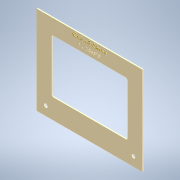
# Autodesk Inventor part: front
Saved by Autodesk Inventor 2022 (Build 260153000, 153)
## iProperties
Created: 2023-08-31
Part Number: front
Material: Generic
Document SubType Name: Modeling
Designer: THK
Density: 1 g/cm^3
Appearance: Red
Author: THK
Autodesk Inventor part; units mm, degrees
ref_plane "YZ Plane" through (0, 0, 0) normal (1, 0, 0) x (0, 1, 0)
ref_plane "XZ Plane" through (0, 0, 0) normal (0, 1, 0) x (-1, 0, 0)
ref_plane "XY Plane" through (0, 0, 0) normal (0, 0, 1) x (1, 0, 0)
sketch "Sketch1" plane through (0, 0, 0) normal (0, 0, 1) x (1, 0, 0)
  line L0 (-264.1156, 220.8859) -> (264.1156, 220.8859)
  line L1 (264.1156, 220.8859) -> (264.1156, -220.8859)
  line L2 (264.1156, -220.8859) -> (-264.1156, -220.8859)
  line L3 (-264.1156, -220.8859) -> (-264.1156, 220.8859)
  line L4 (-264.1156, 220.8859) -> (264.1156, -220.8859) construction
  line L5 (264.1156, 220.8859) -> (-264.1156, -220.8859) construction
  point P0 (0, 0)
  dimension "d0" = 528.2313
  dimension "d1" = 441.7719
  constraints: 12 end point, 2 midpoint, 2 parallel, 1 horizontal, 1 perpendicular
  measures "d0" distance of L1.end L2.end
  measures "d1" distance of L0.end L1.end
extrude "Extrusion1" add sketch "Sketch1" against normal blind 6
sketch "Sketch2" plane through (0, 0, 0) normal (0, 0, 1) x (1, 0, 0)
  line L0 (-181.2094, 146.2703) -> (181.2094, 146.2703)
  line L1 (189.5, 137.9797) -> (189.5, -113.1078)
  line L2 (181.2094, -121.3984) -> (-181.2094, -121.3984)
  line L3 (-189.5, -113.1078) -> (-189.5, 137.9797)
  line L4 (-189.5, 146.2703) -> (189.5, -121.3984) construction
  line L5 (189.5, 146.2703) -> (-189.5, -121.3984) construction
  line L6 (189.5, 105.3059) -> (264.1156, 105.3059) construction
  line L7 (264.1156, 220.8859) -> (264.1156, -220.8859) projected
  line L8 (72.6661, 146.2703) -> (72.6661, 220.8859) construction
  line L9 (-264.1156, 220.8859) -> (264.1156, 220.8859) projected
  arc A0 (-181.2094, 146.2703) -> (-189.5, 137.9797) centre (-181.2094, 137.9797) ccw
  arc A1 (189.5, 137.9797) -> (181.2094, 146.2703) centre (181.2094, 137.9797) ccw
  arc A2 (181.2094, -121.3984) -> (189.5, -113.1078) centre (181.2094, -113.1078) ccw
  arc A3 (-189.5, -113.1078) -> (-181.2094, -121.3984) centre (-181.2094, -113.1078) ccw
  point P0 (0, 0)
  point P1 (0, 12.4359)
  point P2 (0, 12.4359)
  dimension "d4" = 267.6687
  dimension "d5" = 379
  dimension "d6" = 74.6156
  dimension "d7" = 8.2906
  constraints: 16 end point, 12 point on line, 8 point on circle, 8 tangent, 4 centre point, 3 equal radius, 3 midpoint, 2 horizontal, 2 parallel, 2 perpendicular, 1 vertical, 1 vertical alignment
  measures "d4" distance between parallel lines of L2 L0
  measures "d5" distance between parallel lines of L1 L3
  measures "d6" distance between parallel lines of L7 L1
  measures "d7" radius of A0
extrude "Extrusion2" cut sketch "Sketch2" against normal through all
sketch "Sketch3" plane through (0, 0, 0) normal (0, 0, 1) x (1, 0, 0)
  line L0 (-264.1156, -220.8859) -> (-264.1156, 220.8859) construction
  line L1 (-264.1156, -220.8859) -> (-219.1094, -220.8859) construction
  line L2 (-219.1094, -220.8859) -> (-219.1094, -175.8797) construction
  line L3 (-219.1094, -175.8797) -> (-264.1156, -175.8797) construction
  line L4 (-264.1156, -175.8797) -> (-264.1156, -220.8859) construction
  point P0 (0, 0)
  dimension "d10" = 45.0063
  dimension "d11" = 45.0063
  constraints: 8 end point, 2 parallel, 1 coincident, 1 horizontal, 1 perpendicular
  measures "d10" distance of L3.end L2.end
  measures "d11" distance of L2.end L1.end
hole "Hole1" at (-219.1094, -175.8797, 0) direction (0, 0, -1) diameter 19 end through all
mirror "Mirror1" about plane through (0, 0, 0) normal (1, 0, 0) of "Hole1"
sketch "Sketch4" plane through (0, 0, 0) normal (0, 0, 1) x (1, 0, 0)
  line L0 (-184.2304, 215.2203) -> (184.2304, 215.2203) construction
  line L1 (184.2304, 215.2203) -> (184.2304, 133.9272) construction
  line L2 (184.2304, 133.9272) -> (-184.2304, 133.9272) construction
  line L3 (-184.2304, 133.9272) -> (-184.2304, 215.2203) construction
  spline S0 degree 2 poles (-80.6136, 205.9581) (-79.2403, 205.9581) (-73.7327, 205.7536) (-72.3594, 205.7536) knots 0 0 0 1 2 2 2
  spline S1 degree 2 poles (-72.3594, 205.7536) (-70.2264, 205.7536) (-69.4668, 205.8558) knots 0 0 0 1 1 1
  spline S2 degree 2 poles (-69.4668, 205.8558) (-67.8159, 206.0896) (-66.8663, 206.9661) knots 0 0 0 1 1 1
  spline S3 degree 2 poles (-66.8663, 206.9661) (-67.4653, 204.8916) (-69.8904, 203.7813) knots 0 0 0 1 1 1
  spline S4 degree 2 poles (-69.8904, 203.7813) (-70.8693, 203.3285) (-72.4178, 203.3285) knots 0 0 0 1 1 1
  spline S5 degree 2 poles (-72.4178, 203.3285) (-72.7392, 203.3285) (-75.3105, 203.3869) knots 0 0 0 1 1 1
  line L4 (-75.3105, 203.3869) -> (-78.2177, 203.3869)
  spline S6 degree 2 poles (-78.2177, 203.3869) (-78.5829, 203.3869) (-79.9562, 203.3285) knots 0 0 0 1 1 1
  spline S7 degree 2 poles (-79.9562, 203.3285) (-79.8247, 202.4665) (-78.8459, 201.327) knots 0 0 0 1 1 1
  spline S8 degree 2 poles (-78.8459, 201.327) (-77.3703, 199.6031) (-72.8707, 197.5578) (-70.5479, 197.5578) knots 0 0 0 1 2 2 2
  spline S9 degree 2 poles (-70.5479, 197.5578) (-68.7801, 197.5578) (-64.3389, 198.9895) (-63.0095, 200.0122) knots 0 0 0 1 2 2 2
  spline S10 degree 2 poles (-63.0095, 200.0122) (-63.4624, 199.121) (-64.485, 198.2445) knots 0 0 0 1 1 1
  spline S11 degree 2 poles (-64.485, 198.2445) (-66.092, 196.9004) (-70.4748, 195.3226) (-72.6224, 195.3226) knots 0 0 0 1 2 2 2
  spline S12 degree 2 poles (-72.6224, 195.3226) (-74.1855, 195.3226) (-77.9255, 196.5352) (-79.1088, 197.4848) knots 0 0 0 1 2 2 2
  spline S13 degree 2 poles (-79.1088, 197.4848) (-80.3945, 198.5074) (-82.2498, 201.7507) (-82.5128, 203.4161) knots 0 0 0 1 2 2 2
  spline S14 degree 2 poles (-82.5128, 203.4161) (-83.7984, 203.3577) (-84.2513, 203.3285) knots 0 0 0 1 1 1
  spline S15 degree 2 poles (-84.2513, 203.3285) (-85.1717, 203.2554) (-85.9313, 202.9924) knots 0 0 0 1 1 1
  spline S16 degree 2 poles (-85.9313, 202.9924) (-84.8795, 205.2861) (-82.2644, 205.8851) knots 0 0 0 1 1 1
  spline S17 degree 2 poles (-82.2644, 205.8851) (-81.4463, 209.7419) (-78.9481, 211.9041) knots 0 0 0 1 1 1
  spline S18 degree 2 poles (-78.9481, 211.9041) (-77.1658, 213.4526) (-72.2279, 215.2203) (-69.8174, 215.2203) knots 0 0 0 1 2 2 2
  spline S19 degree 2 poles (-69.8174, 215.2203) (-67.3923, 215.2203) (-65.4638, 214.5045) knots 0 0 0 1 1 1
  spline S20 degree 2 poles (-65.4638, 214.5045) (-62.7758, 213.5403) (-62.7758, 211.5096) knots 0 0 0 1 1 1
  spline S21 degree 2 poles (-62.7758, 211.5096) (-62.7758, 209.8442) (-64.3389, 207.682) knots 0 0 0 1 1 1
  spline S22 degree 2 poles (-64.3389, 207.682) (-64.2805, 209.6104) (-65.9898, 211.8164) (-67.889, 212.43) knots 0 0 0 1 2 2 2
  spline S23 degree 2 poles (-67.889, 212.43) (-69.5544, 212.9559) (-71.4244, 212.9559) knots 0 0 0 1 1 1
  spline S24 degree 2 poles (-71.4244, 212.9559) (-73.4989, 212.9559) (-75.7633, 212.1962) knots 0 0 0 1 1 1
  spline S25 degree 2 poles (-75.7633, 212.1962) (-78.2907, 211.3489) (-80.4529, 208.5732) (-80.6136, 205.9581) knots 0 0 0 1 2 2 2
  line L5 (-59.3718, 207.8719) -> (-57.3703, 208.2371)
  line L6 (-57.3703, 208.2371) -> (-57.9547, 205.1254)
  spline S26 degree 2 poles (-57.9547, 205.1254) (-57.8963, 205.1254) (-57.6918, 205.1254) knots 0 0 0 1 1 1
  spline S27 degree 2 poles (-57.6918, 205.1254) (-57.458, 205.1254) (-57.2681, 205.1254) knots 0 0 0 1 1 1
  line L7 (-57.2681, 205.1254) -> (-56.5815, 205.1254)
  spline S28 degree 2 poles (-56.5815, 205.1254) (-55.1936, 205.1254) (-54.8137, 205.0962) knots 0 0 0 1 1 1
  line L8 (-54.8137, 205.0962) -> (-56.2454, 202.861)
  spline S29 degree 2 poles (-56.2454, 202.861) (-57.2389, 202.9924) (-58.2615, 203.0217) knots 0 0 0 1 1 1
  spline S30 degree 2 poles (-58.2615, 203.0217) (-58.4514, 202.1743) (-58.4514, 201.3124) knots 0 0 0 1 1 1
  spline S31 degree 2 poles (-58.4514, 201.3124) (-58.4514, 200.392) (-57.3265, 199.3255) (-56.3769, 199.3255) knots 0 0 0 1 2 2 2
  spline S32 degree 2 poles (-56.3769, 199.3255) (-55.6026, 199.3255) (-55.0621, 199.4132) knots 0 0 0 1 1 1
  line L9 (-55.0621, 199.4132) -> (-57.5018, 197.6163)
  spline S33 degree 2 poles (-57.5018, 197.6163) (-57.8232, 197.3825) (-58.7728, 197.3825) knots 0 0 0 1 1 1
  spline S34 degree 2 poles (-58.7728, 197.3825) (-59.8247, 197.3825) (-60.4091, 198.2298) knots 0 0 0 1 1 1
  spline S35 degree 2 poles (-60.4091, 198.2298) (-60.9058, 198.9603) (-60.9058, 200.0706) knots 0 0 0 1 1 1
  spline S36 degree 2 poles (-60.9058, 200.0706) (-60.9058, 201.0932) (-60.5113, 203.0655) knots 0 0 0 1 1 1
  spline S37 degree 2 poles (-60.5113, 203.0655) (-61.271, 203.0217) (-62.0891, 202.861) knots 0 0 0 1 1 1
  line L10 (-62.0891, 202.861) -> (-61.0373, 204.9939)
  spline S38 degree 2 poles (-61.0373, 204.9939) (-60.7743, 205.0523) (-60.0584, 205.1254) knots 0 0 0 1 1 1
  spline S39 degree 2 poles (-60.0584, 205.1254) (-59.8539, 205.9727) (-59.3718, 207.8719) knots 0 0 0 1 1 1
  line L11 (-44.821, 200.392) -> (-45.42, 199.048)
  spline S40 degree 2 poles (-45.42, 199.048) (-47.7429, 197.4117) (-49.8758, 197.4117) knots 0 0 0 1 1 1
  spline S41 degree 2 poles (-49.8758, 197.4117) (-51.5267, 197.4117) (-53.718, 199.4716) (-53.718, 201.0932) knots 0 0 0 1 2 2 2
  spline S42 degree 2 poles (-53.718, 201.0932) (-53.718, 202.8025) (-51.775, 204.1027) knots 0 0 0 1 1 1
  spline S43 degree 2 poles (-51.775, 204.1027) (-50.0365, 205.2276) (-48.2104, 205.2276) knots 0 0 0 1 1 1
  spline S44 degree 2 poles (-48.2104, 205.2276) (-46.1359, 205.2276) (-44.9964, 204.1173) knots 0 0 0 1 1 1
  line L12 (-44.9964, 204.1173) -> (-46.7348, 201.736)
  spline S45 degree 2 poles (-46.7348, 201.736) (-47.1585, 202.598) (-48.9847, 203.8106) (-49.905, 203.8106) knots 0 0 0 1 2 2 2
  spline S46 degree 2 poles (-49.905, 203.8106) (-51.8773, 203.8106) (-51.8773, 202.2035) knots 0 0 0 1 1 1
  spline S47 degree 2 poles (-51.8773, 202.2035) (-51.8773, 201.0786) (-50.6939, 200.2897) knots 0 0 0 1 1 1
  spline S48 degree 2 poles (-50.6939, 200.2897) (-49.6421, 199.5739) (-48.4587, 199.5739) knots 0 0 0 1 1 1
  spline S49 degree 2 poles (-48.4587, 199.5739) (-46.7056, 199.5739) (-44.821, 200.392) knots 0 0 0 1 1 1
  line L13 (-40.9788, 211.159) -> (-38.13, 211.7872)
  spline S50 degree 2 poles (-38.13, 211.7872) (-39.2988, 208.1787) (-40.8473, 200.6258) knots 0 0 0 1 1 1
  spline S51 degree 2 poles (-40.8473, 200.6258) (-39.8685, 201.8383) (-38.5829, 203.1824) knots 0 0 0 1 1 1
  spline S52 degree 2 poles (-38.5829, 203.1824) (-38.057, 203.7229) (-37.3703, 204.4095) knots 0 0 0 1 1 1
  spline S53 degree 2 poles (-37.3703, 204.4095) (-36.523, 205.1254) (-35.8656, 205.1254) knots 0 0 0 1 1 1
  spline S54 degree 2 poles (-35.8656, 205.1254) (-34.653, 205.1254) (-34.653, 204.2781) knots 0 0 0 1 1 1
  spline S55 degree 2 poles (-34.653, 204.2781) (-34.7115, 204.0735) (-34.9014, 202.8317) knots 0 0 0 1 1 1
  spline S56 degree 2 poles (-34.9014, 202.8317) (-35.1059, 201.4877) (-35.1059, 200.3043) knots 0 0 0 1 1 1
  spline S57 degree 2 poles (-35.1059, 200.3043) (-35.1059, 198.8288) (-33.5573, 198.2298) knots 0 0 0 1 1 1
  line L14 (-33.5573, 198.2298) -> (-36.5084, 197.2802)
  spline S58 degree 2 poles (-36.5084, 197.2802) (-37.6918, 198.0399) (-37.6918, 200.0706) knots 0 0 0 1 1 1
  spline S59 degree 2 poles (-37.6918, 200.0706) (-37.6918, 200.2751) (-37.5603, 201.6776) (-37.5603, 201.8675) knots 0 0 0 1 2 2 2
  spline S60 degree 2 poles (-37.5603, 201.8675) (-37.5603, 202.4373) (-37.7648, 202.4373) knots 0 0 0 1 1 1
  spline S61 degree 2 poles (-37.7648, 202.4373) (-38.0862, 202.4373) (-38.5099, 202.0428) knots 0 0 0 1 1 1
  spline S62 degree 2 poles (-38.5099, 202.0428) (-40.2922, 200.3628) (-41.8262, 197.9815) knots 0 0 0 1 1 1
  line L15 (-41.8262, 197.9815) -> (-43.6669, 197.3825)
  line L16 (-43.6669, 197.3825) -> (-40.9788, 211.159)
  line L17 (3.9299, 214.9574) -> (1.4317, 203.6937)
  line L18 (1.4317, 203.6937) -> (3.9299, 203.6937)
  line L19 (3.9299, 203.6937) -> (2.5858, 201.59)
  line L20 (2.5858, 201.59) -> (0.9496, 201.59)
  line L21 (0.9496, 201.59) -> (0.2191, 198.2737)
  line L22 (0.2191, 198.2737) -> (-1.5924, 197.3825)
  spline S63 degree 2 poles (-1.5924, 197.3825) (-3.8861, 200.3628) (-7.6844, 201.59) knots 0 0 0 1 1 1
  spline S64 degree 2 poles (-7.6844, 201.59) (-8.7363, 199.9683) (-10.4748, 199.1064) knots 0 0 0 1 1 1
  spline S65 degree 2 poles (-10.4748, 199.1064) (-13.0899, 197.8354) (-15.851, 197.8354) knots 0 0 0 1 1 1
  spline S66 degree 2 poles (-15.851, 197.8354) (-17.7502, 197.8354) (-20.0584, 198.7558) knots 0 0 0 1 1 1
  spline S67 degree 2 poles (-20.0584, 198.7558) (-22.5128, 199.7346) (-22.5128, 201.4439) knots 0 0 0 1 1 1
  spline S68 degree 2 poles (-22.5128, 201.4439) (-22.5128, 203.4892) (-20.3068, 204.7017) knots 0 0 0 1 1 1
  spline S69 degree 2 poles (-20.3068, 204.7017) (-18.4806, 205.6805) (-16.2454, 205.6805) knots 0 0 0 1 1 1
  spline S70 degree 2 poles (-16.2454, 205.6805) (-12.7684, 205.6805) (-10.7378, 203.9128) knots 0 0 0 1 1 1
  spline S71 degree 2 poles (-10.7378, 203.9128) (-12.7392, 204.1466) (-14.9744, 204.1466) knots 0 0 0 1 1 1
  spline S72 degree 2 poles (-14.9744, 204.1466) (-18.3199, 204.1466) (-20.0877, 203.0947) knots 0 0 0 1 1 1
  spline S73 degree 2 poles (-20.0877, 203.0947) (-20.5698, 202.8025) (-20.5698, 202.598) knots 0 0 0 1 1 1
  spline S74 degree 2 poles (-20.5698, 202.598) (-20.5698, 201.8383) (-18.4806, 201.1225) knots 0 0 0 1 1 1
  spline S75 degree 2 poles (-18.4806, 201.1225) (-15.4565, 200.0998) (-13.2213, 200.0998) knots 0 0 0 1 1 1
  spline S76 degree 2 poles (-13.2213, 200.0998) (-9.6567, 200.0998) (-9.233, 201.59) knots 0 0 0 1 1 1
  line L23 (-9.233, 201.59) -> (-10.84, 201.59)
  line L24 (-10.84, 201.59) -> (-9.4814, 203.6937)
  line L25 (-9.4814, 203.6937) -> (-7.027, 203.6937)
  spline S77 degree 2 poles (-7.027, 203.6937) (-5.3178, 209.4205) (-3.4916, 211.8748) knots 0 0 0 1 1 1
  spline S78 degree 2 poles (-3.4916, 211.8748) (-2.1037, 213.774) (-0.2338, 214.4022) knots 0 0 0 1 1 1
  spline S79 degree 2 poles (-0.2338, 214.4022) (1.0957, 214.8551) (3.9299, 214.9574) knots 0 0 0 1 1 1
  line L26 (-5.756, 203.6937) -> (-0.599, 203.6937)
  line L27 (-0.599, 203.6937) -> (1.1103, 212.2108)
  spline S80 degree 2 poles (1.1103, 212.2108) (-3.5793, 211.5534) (-5.756, 203.6937) knots 0 0 0 1 1 1
  line L28 (-1.4901, 199.2233) -> (-1.0226, 201.59)
  line L29 (-1.0226, 201.59) -> (-4.5727, 201.59)
  line L30 (-4.5727, 201.59) -> (-2.9949, 200.4943)
  spline S81 degree 2 poles (-2.9949, 200.4943) (-2.3813, 200.0706) (-1.4901, 199.2233) knots 0 0 0 1 1 1
  spline S82 degree 2 poles (16.9905, 203.5768) (16.786, 202.934) (16.786, 202.3642) knots 0 0 0 1 1 1
  spline S83 degree 2 poles (16.786, 202.3642) (16.786, 199.8953) (20.1023, 198.7558) knots 0 0 0 1 1 1
  spline S84 degree 2 poles (20.1023, 198.7558) (22.4105, 197.9669) (25.4784, 197.9669) knots 0 0 0 1 1 1
  spline S85 degree 2 poles (25.4784, 197.9669) (27.889, 197.9669) (29.7151, 198.4636) knots 0 0 0 1 1 1
  spline S86 degree 2 poles (29.7151, 198.4636) (32.6077, 199.2525) (32.6077, 201.0202) knots 0 0 0 1 1 1
  spline S87 degree 2 poles (32.6077, 201.0202) (32.6077, 201.9698) (31.8919, 202.7587) knots 0 0 0 1 1 1
  spline S88 degree 2 poles (31.8919, 202.7587) (31.2637, 203.4745) (30.3141, 203.8106) knots 0 0 0 1 1 1
  spline S89 degree 2 poles (30.3141, 203.8106) (29.16, 204.205) (26.1505, 205.2569) knots 0 0 0 1 1 1
  spline S90 degree 2 poles (26.1505, 205.2569) (23.886, 206.075) (22.8342, 206.7908) knots 0 0 0 1 1 1
  spline S91 degree 2 poles (22.8342, 206.7908) (21.0226, 208.0034) (21.0226, 209.7127) knots 0 0 0 1 1 1
  spline S92 degree 2 poles (21.0226, 209.7127) (21.0226, 211.3489) (22.8926, 212.8829) knots 0 0 0 1 1 1
  spline S93 degree 2 poles (22.8926, 212.8829) (24.4266, 214.11) (26.2966, 214.6944) knots 0 0 0 1 1 1
  spline S94 degree 2 poles (26.2966, 214.6944) (27.9766, 215.2203) (29.6567, 215.2203) knots 0 0 0 1 1 1
  spline S95 degree 2 poles (29.6567, 215.2203) (32.0818, 215.2203) (34.054, 214.2123) knots 0 0 0 1 1 1
  spline S96 degree 2 poles (34.054, 214.2123) (35.5588, 213.4526) (35.5588, 212.503) knots 0 0 0 1 1 1
  spline S97 degree 2 poles (35.5588, 212.503) (35.5588, 211.5242) (34.8576, 210.896) knots 0 0 0 1 1 1
  line L31 (34.8576, 210.896) -> (32.7684, 209.0553)
  spline S98 degree 2 poles (32.7684, 209.0553) (33.0022, 209.8149) (33.0022, 210.4724) knots 0 0 0 1 1 1
  line L32 (33.0022, 210.4724) -> (33.0022, 210.8376)
  spline S99 degree 2 poles (33.0022, 210.8376) (33.0022, 211.7141) (31.6581, 212.5323) knots 0 0 0 1 1 1
  spline S100 degree 2 poles (31.6581, 212.5323) (29.7882, 213.6864) (27.4945, 213.6864) knots 0 0 0 1 1 1
  spline S101 degree 2 poles (27.4945, 213.6864) (24.4996, 213.6864) (23.3601, 212.0501) knots 0 0 0 1 1 1
  spline S102 degree 2 poles (23.3601, 212.0501) (23.0533, 211.6119) (23.0533, 211.1298) knots 0 0 0 1 1 1
  spline S103 degree 2 poles (23.0533, 211.1298) (23.0533, 209.625) (25.5515, 208.6608) knots 0 0 0 1 1 1
  spline S104 degree 2 poles (25.5515, 208.6608) (26.691, 208.2371) (29.6129, 207.1268) knots 0 0 0 1 1 1
  spline S105 degree 2 poles (29.6129, 207.1268) (31.8773, 206.2649) (32.8269, 205.5783) knots 0 0 0 1 1 1
  spline S106 degree 2 poles (32.8269, 205.5783) (34.5362, 204.3365) (34.5362, 202.6564) knots 0 0 0 1 1 1
  spline S107 degree 2 poles (34.5362, 202.6564) (34.5362, 200.4943) (31.9795, 198.6681) knots 0 0 0 1 1 1
  spline S108 degree 2 poles (31.9795, 198.6681) (28.1373, 195.9362) (22.5274, 195.9362) knots 0 0 0 1 1 1
  spline S109 degree 2 poles (22.5274, 195.9362) (18.6998, 195.9362) (16.3039, 197.514) knots 0 0 0 1 1 1
  spline S110 degree 2 poles (16.3039, 197.514) (14.5946, 198.6535) (14.5946, 200.129) knots 0 0 0 1 1 1
  spline S111 degree 2 poles (14.5946, 200.129) (14.5946, 200.7572) (14.7845, 200.9618) knots 0 0 0 1 1 1
  line L33 (14.7845, 200.9618) -> (16.9905, 203.5768)
  line L34 (37.7356, 211.2613) -> (40.4821, 211.8164)
  spline S112 degree 2 poles (40.4821, 211.8164) (39.6786, 209.0991) (38.7144, 202.8025) knots 0 0 0 1 1 1
  spline S113 degree 2 poles (38.7144, 202.8025) (41.0226, 205.6075) (43.1556, 205.6075) knots 0 0 0 1 1 1
  spline S114 degree 2 poles (43.1556, 205.6075) (44.1052, 205.6075) (44.7626, 205.1838) knots 0 0 0 1 1 1
  spline S115 degree 2 poles (44.7626, 205.1838) (45.5661, 204.7163) (45.5661, 203.8106) knots 0 0 0 1 1 1
  spline S116 degree 2 poles (45.5661, 203.8106) (45.5661, 202.7149) (44.2221, 201.7653) knots 0 0 0 1 1 1
  spline S117 degree 2 poles (44.2221, 201.7653) (43.6377, 201.3416) (41.9284, 200.5527) knots 0 0 0 1 1 1
  spline S118 degree 2 poles (41.9284, 200.5527) (43.5354, 199.8953) (46.3258, 199.5155) knots 0 0 0 1 1 1
  line L35 (46.3258, 199.5155) -> (44.1052, 197.3095)
  spline S119 degree 2 poles (44.1052, 197.3095) (40.9496, 197.777) (38.4806, 199.5739) knots 0 0 0 1 1 1
  line L36 (38.4806, 199.5739) -> (39.8977, 201.4146)
  line L37 (39.8977, 201.4146) -> (41.7677, 201.4146)
  spline S120 degree 2 poles (41.7677, 201.4146) (42.7173, 201.4146) (42.7173, 202.4373) knots 0 0 0 1 1 1
  spline S121 degree 2 poles (42.7173, 202.4373) (42.7173, 202.8902) (42.0307, 203.606) (41.5778, 203.606) knots 0 0 0 1 2 2 2
  spline S122 degree 2 poles (41.5778, 203.606) (39.8977, 203.606) (38.9189, 201.4731) knots 0 0 0 1 1 1
  spline S123 degree 2 poles (38.9189, 201.4731) (38.4514, 200.3043) (37.5018, 197.9669) knots 0 0 0 1 1 1
  line L38 (37.5018, 197.9669) -> (35.6026, 197.3825)
  line L39 (35.6026, 197.3825) -> (37.7356, 211.2613)
  line L40 (49.6421, 201.2832) -> (50.1388, 202.4957)
  spline S124 degree 2 poles (50.1388, 202.4957) (51.3221, 202.262) (52.374, 202.262) knots 0 0 0 1 1 1
  spline S125 degree 2 poles (52.374, 202.262) (52.8707, 202.262) (52.8707, 202.7295) knots 0 0 0 1 1 1
  spline S126 degree 2 poles (52.8707, 202.7295) (52.8707, 203.8252) (51.2491, 203.8252) knots 0 0 0 1 1 1
  spline S127 degree 2 poles (51.2491, 203.8252) (49.2914, 203.8252) (49.2914, 202.0721) knots 0 0 0 1 1 1
  spline S128 degree 2 poles (49.2914, 202.0721) (49.2914, 201.2978) (50.0073, 200.6258) knots 0 0 0 1 1 1
  spline S129 degree 2 poles (50.0073, 200.6258) (50.6355, 199.9976) (51.4244, 199.7784) knots 0 0 0 1 1 1
  spline S130 degree 2 poles (51.4244, 199.7784) (51.8188, 199.6762) (52.5639, 199.6762) knots 0 0 0 1 1 1
  spline S131 degree 2 poles (52.5639, 199.6762) (54.1125, 199.6762) (56.2746, 200.465) knots 0 0 0 1 1 1
  line L41 (56.2746, 200.465) -> (55.8072, 199.0918)
  spline S132 degree 2 poles (55.8072, 199.0918) (53.3236, 197.4117) (50.8546, 197.4117) knots 0 0 0 1 1 1
  spline S133 degree 2 poles (50.8546, 197.4117) (49.4521, 197.4117) (47.4507, 199.2525) (47.4507, 200.655) knots 0 0 0 1 2 2 2
  spline S134 degree 2 poles (47.4507, 200.655) (47.4507, 202.4373) (48.4733, 203.5184) knots 0 0 0 1 1 1
  spline S135 degree 2 poles (48.4733, 203.5184) (50.241, 205.3591) (52.8707, 205.3591) knots 0 0 0 1 1 1
  spline S136 degree 2 poles (52.8707, 205.3591) (54.0102, 205.3591) (54.8576, 204.9647) knots 0 0 0 1 1 1
  spline S137 degree 2 poles (54.8576, 204.9647) (55.9532, 204.4388) (55.9532, 203.4307) knots 0 0 0 1 1 1
  spline S138 degree 2 poles (55.9532, 203.4307) (55.9532, 202.1159) (54.244, 201.5169) knots 0 0 0 1 1 1
  spline S139 degree 2 poles (54.244, 201.5169) (53.0606, 201.0932) (51.4244, 201.0932) knots 0 0 0 1 1 1
  spline S140 degree 2 poles (51.4244, 201.0932) (50.4748, 201.0932) (49.6421, 201.2832) knots 0 0 0 1 1 1
  line L42 (60.1315, 207.8719) -> (62.1329, 208.2371)
  line L43 (62.1329, 208.2371) -> (61.5486, 205.1254)
  spline S141 degree 2 poles (61.5486, 205.1254) (61.607, 205.1254) (61.8115, 205.1254) knots 0 0 0 1 1 1
  spline S142 degree 2 poles (61.8115, 205.1254) (62.0453, 205.1254) (62.2352, 205.1254) knots 0 0 0 1 1 1
  line L44 (62.2352, 205.1254) -> (62.9218, 205.1254)
  spline S143 degree 2 poles (62.9218, 205.1254) (64.3097, 205.1254) (64.6895, 205.0962) knots 0 0 0 1 1 1
  line L45 (64.6895, 205.0962) -> (63.2578, 202.861)
  spline S144 degree 2 poles (63.2578, 202.861) (62.2644, 202.9924) (61.2418, 203.0217) knots 0 0 0 1 1 1
  spline S145 degree 2 poles (61.2418, 203.0217) (61.0519, 202.1743) (61.0519, 201.3124) knots 0 0 0 1 1 1
  spline S146 degree 2 poles (61.0519, 201.3124) (61.0519, 200.392) (62.1768, 199.3255) (63.1264, 199.3255) knots 0 0 0 1 2 2 2
  spline S147 degree 2 poles (63.1264, 199.3255) (63.9007, 199.3255) (64.4412, 199.4132) knots 0 0 0 1 1 1
  line L46 (64.4412, 199.4132) -> (62.0015, 197.6163)
  spline S148 degree 2 poles (62.0015, 197.6163) (61.6801, 197.3825) (60.7305, 197.3825) knots 0 0 0 1 1 1
  spline S149 degree 2 poles (60.7305, 197.3825) (59.6786, 197.3825) (59.0942, 198.2298) knots 0 0 0 1 1 1
  spline S150 degree 2 poles (59.0942, 198.2298) (58.5975, 198.9603) (58.5975, 200.0706) knots 0 0 0 1 1 1
  spline S151 degree 2 poles (58.5975, 200.0706) (58.5975, 201.0932) (58.992, 203.0655) knots 0 0 0 1 1 1
  spline S152 degree 2 poles (58.992, 203.0655) (58.2323, 203.0217) (57.4142, 202.861) knots 0 0 0 1 1 1
  line L47 (57.4142, 202.861) -> (58.466, 204.9939)
  spline S153 degree 2 poles (58.466, 204.9939) (58.729, 205.0523) (59.4448, 205.1254) knots 0 0 0 1 1 1
  spline S154 degree 2 poles (59.4448, 205.1254) (59.6494, 205.9727) (60.1315, 207.8719) knots 0 0 0 1 1 1
  line L48 (74.6822, 200.392) -> (74.0833, 199.048)
  spline S155 degree 2 poles (74.0833, 199.048) (71.7604, 197.4117) (69.6275, 197.4117) knots 0 0 0 1 1 1
  spline S156 degree 2 poles (69.6275, 197.4117) (67.9766, 197.4117) (65.7852, 199.4716) (65.7852, 201.0932) knots 0 0 0 1 2 2 2
  spline S157 degree 2 poles (65.7852, 201.0932) (65.7852, 202.8025) (67.7283, 204.1027) knots 0 0 0 1 1 1
  spline S158 degree 2 poles (67.7283, 204.1027) (69.4668, 205.2276) (71.2929, 205.2276) knots 0 0 0 1 1 1
  spline S159 degree 2 poles (71.2929, 205.2276) (73.3674, 205.2276) (74.5069, 204.1173) knots 0 0 0 1 1 1
  line L49 (74.5069, 204.1173) -> (72.7684, 201.736)
  spline S160 degree 2 poles (72.7684, 201.736) (72.3448, 202.598) (70.5186, 203.8106) (69.5982, 203.8106) knots 0 0 0 1 2 2 2
  spline S161 degree 2 poles (69.5982, 203.8106) (67.626, 203.8106) (67.626, 202.2035) knots 0 0 0 1 1 1
  spline S162 degree 2 poles (67.626, 202.2035) (67.626, 201.0786) (68.8093, 200.2897) knots 0 0 0 1 1 1
  spline S163 degree 2 poles (68.8093, 200.2897) (69.8612, 199.5739) (71.0446, 199.5739) knots 0 0 0 1 1 1
  spline S164 degree 2 poles (71.0446, 199.5739) (72.7977, 199.5739) (74.6822, 200.392) knots 0 0 0 1 1 1
  line L50 (78.5245, 211.159) -> (81.3733, 211.7872)
  spline S165 degree 2 poles (81.3733, 211.7872) (80.2045, 208.1787) (78.6559, 200.6258) knots 0 0 0 1 1 1
  spline S166 degree 2 poles (78.6559, 200.6258) (79.6348, 201.8383) (80.9204, 203.1824) knots 0 0 0 1 1 1
  spline S167 degree 2 poles (80.9204, 203.1824) (81.4463, 203.7229) (82.1329, 204.4095) knots 0 0 0 1 1 1
  spline S168 degree 2 poles (82.1329, 204.4095) (82.9803, 205.1254) (83.6377, 205.1254) knots 0 0 0 1 1 1
  spline S169 degree 2 poles (83.6377, 205.1254) (84.8502, 205.1254) (84.8502, 204.2781) knots 0 0 0 1 1 1
  spline S170 degree 2 poles (84.8502, 204.2781) (84.7918, 204.0735) (84.6019, 202.8317) knots 0 0 0 1 1 1
  spline S171 degree 2 poles (84.6019, 202.8317) (84.3974, 201.4877) (84.3974, 200.3043) knots 0 0 0 1 1 1
  spline S172 degree 2 poles (84.3974, 200.3043) (84.3974, 198.8288) (85.9459, 198.2298) knots 0 0 0 1 1 1
  line L51 (85.9459, 198.2298) -> (82.9949, 197.2802)
  spline S173 degree 2 poles (82.9949, 197.2802) (81.8115, 198.0399) (81.8115, 200.0706) knots 0 0 0 1 1 1
  spline S174 degree 2 poles (81.8115, 200.0706) (81.8115, 200.2751) (81.943, 201.6776) (81.943, 201.8675) knots 0 0 0 1 2 2 2
  spline S175 degree 2 poles (81.943, 201.8675) (81.943, 202.4373) (81.7385, 202.4373) knots 0 0 0 1 1 1
  spline S176 degree 2 poles (81.7385, 202.4373) (81.4171, 202.4373) (80.9934, 202.0428) knots 0 0 0 1 1 1
  spline S177 degree 2 poles (80.9934, 202.0428) (79.2111, 200.3628) (77.6771, 197.9815) knots 0 0 0 1 1 1
  line L52 (77.6771, 197.9815) -> (75.8364, 197.3825)
  line L53 (75.8364, 197.3825) -> (78.5245, 211.159)
  line L54 (-48.9262, 178.5052) -> (-47.5091, 178.5052)
  line L55 (-47.5091, 178.5052) -> (-50.1388, 164.3635)
  line L56 (-50.1388, 164.3635) -> (-51.9795, 163.8376)
  line L57 (-51.9795, 163.8376) -> (-50.4748, 175.5834)
  spline S178 degree 2 poles (-50.4748, 175.5834) (-51.8188, 174.6338) (-53.3528, 174.1955) knots 0 0 0 1 1 1
  line L58 (-53.3528, 174.1955) -> (-53.3528, 175.2182)
  spline S179 degree 2 poles (-53.3528, 175.2182) (-50.6939, 176.4307) (-48.9262, 178.5052) knots 0 0 0 1 1 1
  line L59 (-36.4354, 165.3424) -> (-34.8283, 166.7156)
  line L60 (-34.8283, 166.7156) -> (-33.5573, 165.1817)
  line L61 (-33.5573, 165.1817) -> (-35.0913, 163.8376)
  line L62 (-35.0913, 163.8376) -> (-36.4354, 165.3424)
  line L63 (-35.3835, 168.9947) -> (-33.7765, 170.3679)
  line L64 (-33.7765, 170.3679) -> (-32.5055, 168.8486)
  line L65 (-32.5055, 168.8486) -> (-34.0394, 167.5045)
  line L66 (-34.0394, 167.5045) -> (-35.3835, 168.9947)
  line L67 (-17.7648, 174.0348) -> (-19.3718, 172.8515)
  spline S180 degree 2 poles (-19.3718, 172.8515) (-19.737, 173.5819) (-19.737, 174.1955) knots 0 0 0 1 1 1
  spline S181 degree 2 poles (-19.737, 174.1955) (-19.737, 176.0655) (-18.0278, 177.3511) knots 0 0 0 1 1 1
  spline S182 degree 2 poles (-18.0278, 177.3511) (-16.4646, 178.5637) (-14.5508, 178.5637) knots 0 0 0 1 1 1
  spline S183 degree 2 poles (-14.5508, 178.5637) (-12.8853, 178.5637) (-11.8042, 177.804) knots 0 0 0 1 1 1
  spline S184 degree 2 poles (-11.8042, 177.804) (-10.5625, 176.9275) (-10.5625, 175.3204) knots 0 0 0 1 1 1
  spline S185 degree 2 poles (-10.5625, 175.3204) (-10.5625, 173.4797) (-11.5851, 171.9019) knots 0 0 0 1 1 1
  spline S186 degree 2 poles (-11.5851, 171.9019) (-12.3302, 170.7916) (-14.0541, 169.1846) knots 0 0 0 1 1 1
  spline S187 degree 2 poles (-14.0541, 169.1846) (-14.8137, 168.4979) (-16.7714, 166.6864) knots 0 0 0 1 1 1
  spline S188 degree 2 poles (-16.7714, 166.6864) (-16.1286, 166.6864) (-13.6012, 166.4673) (-12.973, 166.4673) knots 0 0 0 1 2 2 2
  spline S189 degree 2 poles (-12.973, 166.4673) (-12.1256, 166.4673) (-11.3952, 166.628) knots 0 0 0 1 1 1
  line L68 (-11.3952, 166.628) -> (-13.4259, 163.8376)
  line L69 (-13.4259, 163.8376) -> (-18.3199, 164.0714)
  spline S190 degree 2 poles (-18.3199, 164.0714) (-20.5552, 164.0714) (-21.4025, 163.8376) knots 0 0 0 1 1 1
  line L70 (-21.4025, 163.8376) -> (-19.5033, 166.628)
  spline S191 degree 2 poles (-19.5033, 166.628) (-19.1381, 166.6864) (-18.393, 166.7156) knots 0 0 0 1 1 1
  spline S192 degree 2 poles (-18.393, 166.7156) (-17.2681, 167.7383) (-16.1286, 168.7317) knots 0 0 0 1 1 1
  spline S193 degree 2 poles (-16.1286, 168.7317) (-14.7845, 170.0319) (-14.1563, 171.0253) knots 0 0 0 1 1 1
  spline S194 degree 2 poles (-14.1563, 171.0253) (-13.309, 172.3694) (-13.309, 173.8449) knots 0 0 0 1 1 1
  spline S195 degree 2 poles (-13.309, 173.8449) (-13.309, 175.5104) (-13.8641, 176.2993) knots 0 0 0 1 1 1
  spline S196 degree 2 poles (-13.8641, 176.2993) (-14.1271, 176.6645) (-15.2082, 177.2489) (-15.6903, 177.2489) knots 0 0 0 1 2 2 2
  spline S197 degree 2 poles (-15.6903, 177.2489) (-16.6837, 177.2489) (-17.3119, 176.7668) knots 0 0 0 1 1 1
  spline S198 degree 2 poles (-17.3119, 176.7668) (-18.0278, 176.2408) (-18.0278, 175.2912) knots 0 0 0 1 1 1
  spline S199 degree 2 poles (-18.0278, 175.2912) (-18.0278, 174.5608) (-17.7648, 174.0348) knots 0 0 0 1 1 1
  line L71 (-8.7655, 165.2401) -> (-6.7348, 166.7156)
  spline S200 degree 2 poles (-6.7348, 166.7156) (-6.2089, 166.0582) (-6.2089, 165.1524) knots 0 0 0 1 1 1
  spline S201 degree 2 poles (-6.2089, 165.1524) (-6.2089, 163.9107) (-8.2688, 161.617) (-9.4814, 161.3833) knots 0 0 0 1 2 2 2
  spline S202 degree 2 poles (-9.4814, 161.3833) (-8.4003, 162.9464) (-8.4003, 163.8084) knots 0 0 0 1 1 1
  spline S203 degree 2 poles (-8.4003, 163.8084) (-8.4003, 164.5535) (-8.7655, 165.2401) knots 0 0 0 1 1 1
  line L72 (-1.2856, 170.4994) -> (0.4821, 172.9537)
  line L73 (0.4821, 172.9537) -> (0.6428, 172.9537)
  spline S204 degree 2 poles (0.6428, 172.9537) (1.3002, 172.9537) (2.1914, 172.72) knots 0 0 0 1 1 1
  spline S205 degree 2 poles (2.1914, 172.72) (2.878, 173.5527) (2.878, 174.4293) knots 0 0 0 1 1 1
  spline S206 degree 2 poles (2.878, 174.4293) (2.878, 177.1028) (0.6136, 177.1028) knots 0 0 0 1 1 1
  spline S207 degree 2 poles (0.6136, 177.1028) (-1.5632, 177.1028) (-2.8926, 175.2182) knots 0 0 0 1 1 1
  line L74 (-2.8926, 175.2182) -> (-2.8342, 177.2489)
  spline S208 degree 2 poles (-2.8342, 177.2489) (-0.7451, 178.6367) (1.6216, 178.6367) knots 0 0 0 1 1 1
  spline S209 degree 2 poles (1.6216, 178.6367) (4.0175, 178.6367) (5.011, 176.9713) knots 0 0 0 1 1 1
  spline S210 degree 2 poles (5.011, 176.9713) (5.3324, 176.4453) (5.3324, 176.0071) knots 0 0 0 1 1 1
  spline S211 degree 2 poles (5.3324, 176.0071) (5.3324, 173.9472) (3.4332, 172.3109) knots 0 0 0 1 1 1
  spline S212 degree 2 poles (3.4332, 172.3109) (5.7414, 171.2591) (5.7414, 169.4183) knots 0 0 0 1 1 1
  spline S213 degree 2 poles (5.7414, 169.4183) (5.7414, 166.9494) (3.9299, 165.3716) knots 0 0 0 1 1 1
  spline S214 degree 2 poles (3.9299, 165.3716) (2.2206, 163.8376) (-0.2776, 163.8376) knots 0 0 0 1 1 1
  spline S215 degree 2 poles (-0.2776, 163.8376) (-3.1556, 163.8376) (-5.0986, 166.2043) knots 0 0 0 1 1 1
  line L75 (-5.0986, 166.2043) -> (-2.8342, 168.8924)
  spline S216 degree 2 poles (-2.8342, 168.8924) (-2.469, 167.5337) (-1.2564, 166.4234) knots 0 0 0 1 1 1
  spline S217 degree 2 poles (-1.2564, 166.4234) (0.0292, 165.2401) (1.3733, 165.2401) knots 0 0 0 1 1 1
  spline S218 degree 2 poles (1.3733, 165.2401) (3.4039, 165.2401) (3.4039, 167.3438) knots 0 0 0 1 1 1
  spline S219 degree 2 poles (3.4039, 167.3438) (3.4039, 168.98) (1.271, 170.6601) (-0.3798, 170.6601) knots 0 0 0 1 2 2 2
  spline S220 degree 2 poles (-0.3798, 170.6601) (-0.599, 170.6601) (-1.2856, 170.4994) knots 0 0 0 1 1 1
  line L76 (12.2425, 173.4505) -> (12.6077, 173.4505)
  spline S221 degree 2 poles (12.6077, 173.4505) (14.7261, 173.4505) (15.9825, 172.457) knots 0 0 0 1 1 1
  spline S222 degree 2 poles (15.9825, 172.457) (17.385, 171.376) (17.385, 169.3161) knots 0 0 0 1 1 1
  spline S223 degree 2 poles (17.385, 169.3161) (17.385, 168.3665) (16.3623, 166.1897) (15.588, 165.4446) knots 0 0 0 1 2 2 2
  spline S224 degree 2 poles (15.588, 165.4446) (13.9518, 163.8668) (11.4244, 163.8668) knots 0 0 0 1 1 1
  spline S225 degree 2 poles (11.4244, 163.8668) (9.3791, 163.8668) (8.1081, 165.3716) knots 0 0 0 1 1 1
  spline S226 degree 2 poles (8.1081, 165.3716) (6.8955, 166.7594) (6.8955, 168.8486) knots 0 0 0 1 1 1
  spline S227 degree 2 poles (6.8955, 168.8486) (6.8955, 172.5593) (10.5332, 175.4811) knots 0 0 0 1 1 1
  spline S228 degree 2 poles (10.5332, 175.4811) (13.908, 178.1985) (17.7502, 178.4322) knots 0 0 0 1 1 1
  line L77 (17.7502, 178.4322) -> (16.3477, 176.4015)
  line L78 (16.3477, 176.4015) -> (16.0701, 176.4015)
  spline S229 degree 2 poles (16.0701, 176.4015) (12.4616, 176.4015) (10.4748, 173.7426) knots 0 0 0 1 1 1
  spline S230 degree 2 poles (10.4748, 173.7426) (9.3499, 172.2233) (9.3499, 170.4556) knots 0 0 0 1 1 1
  spline S231 degree 2 poles (9.3499, 170.4556) (9.3499, 168.5126) (10.5332, 167.1831) knots 0 0 0 1 1 1
  spline S232 degree 2 poles (10.5332, 167.1831) (11.7458, 165.7952) (13.6742, 165.7952) knots 0 0 0 1 1 1
  spline S233 degree 2 poles (13.6742, 165.7952) (14.4047, 165.7952) (15.6465, 166.7887) (15.6465, 167.4753) knots 0 0 0 1 2 2 2
  spline S234 degree 2 poles (15.6465, 167.4753) (15.6465, 169.0239) (14.1709, 170.0027) knots 0 0 0 1 1 1
  spline S235 degree 2 poles (14.1709, 170.0027) (12.9291, 170.8208) (11.2491, 170.8208) knots 0 0 0 1 1 1
  spline S236 degree 2 poles (11.2491, 170.8208) (10.9861, 170.8208) (10.2995, 170.7624) knots 0 0 0 1 1 1
  line L79 (10.2995, 170.7624) -> (12.2425, 173.4505)
  spline S237 degree 2 poles (29.3499, 168.7171) (29.3499, 166.6864) (25.9021, 163.8376) (23.9007, 163.8376) knots 0 0 0 1 2 2 2
  spline S238 degree 2 poles (23.9007, 163.8376) (21.8992, 163.8376) (20.5259, 164.6849) knots 0 0 0 1 1 1
  spline S239 degree 2 poles (20.5259, 164.6849) (18.8897, 165.6784) (18.8897, 167.5776) knots 0 0 0 1 1 1
  spline S240 degree 2 poles (18.8897, 167.5776) (18.8897, 170.0319) (22.5274, 171.449) knots 0 0 0 1 1 1
  spline S241 degree 2 poles (22.5274, 171.449) (21.2856, 172.4716) (21.2856, 174.1663) knots 0 0 0 1 1 1
  spline S242 degree 2 poles (21.2856, 174.1663) (21.2856, 176.1386) (22.8196, 177.4096) knots 0 0 0 1 1 1
  spline S243 degree 2 poles (22.8196, 177.4096) (24.2659, 178.5637) (26.2966, 178.5637) knots 0 0 0 1 1 1
  spline S244 degree 2 poles (26.2966, 178.5637) (27.6406, 178.5637) (28.5756, 177.8478) knots 0 0 0 1 1 1
  spline S245 degree 2 poles (28.5756, 177.8478) (29.5836, 177.0589) (29.5836, 175.7441) knots 0 0 0 1 1 1
  spline S246 degree 2 poles (29.5836, 175.7441) (29.5836, 173.9033) (26.954, 172.1356) knots 0 0 0 1 1 1
  spline S247 degree 2 poles (26.954, 172.1356) (28.1373, 171.4052) (28.6633, 170.7624) knots 0 0 0 1 1 1
  spline S248 degree 2 poles (28.6633, 170.7624) (29.3499, 169.9004) (29.3499, 168.7171) knots 0 0 0 1 1 1
  spline S249 degree 2 poles (23.1118, 171.0546) (21.4463, 170.3971) (21.4463, 168.9508) knots 0 0 0 1 1 1
  spline S250 degree 2 poles (21.4463, 168.9508) (21.4463, 167.5337) (23.8422, 165.3716) (25.2593, 165.3716) knots 0 0 0 1 2 2 2
  spline S251 degree 2 poles (25.2593, 165.3716) (27.3192, 165.3716) (27.3192, 167.1539) knots 0 0 0 1 1 1
  spline S252 degree 2 poles (27.3192, 167.1539) (27.3192, 168.1035) (26.4719, 168.9216) knots 0 0 0 1 1 1
  spline S253 degree 2 poles (26.4719, 168.9216) (26.0044, 169.4037) (24.7918, 170.105) knots 0 0 0 1 1 1
  spline S254 degree 2 poles (24.7918, 170.105) (24.2951, 170.3971) (23.1118, 171.0546) knots 0 0 0 1 1 1
  spline S255 degree 2 poles (26.2381, 172.5885) (27.3192, 173.4505) (27.3192, 174.7215) knots 0 0 0 1 1 1
  spline S256 degree 2 poles (27.3192, 174.7215) (27.3192, 177.4096) (24.9525, 177.4096) knots 0 0 0 1 1 1
  spline S257 degree 2 poles (24.9525, 177.4096) (23.3163, 177.4096) (23.3163, 175.8756) knots 0 0 0 1 1 1
  spline S258 degree 2 poles (23.3163, 175.8756) (23.3163, 174.7507) (24.2951, 173.8741) knots 0 0 0 1 1 1
  spline S259 degree 2 poles (24.2951, 173.8741) (24.7626, 173.4505) (26.2381, 172.5885) knots 0 0 0 1 1 1
  line L80 (30.767, 175.5104) -> (32.4763, 178.2715)
  spline S260 degree 2 poles (32.4763, 178.2715) (33.0022, 178.4614) (33.908, 178.4614) knots 0 0 0 1 1 1
  spline S261 degree 2 poles (33.908, 178.4614) (34.5654, 178.4614) (37.195, 178.1692) (37.8524, 178.1692) knots 0 0 0 1 2 2 2
  spline S262 degree 2 poles (37.8524, 178.1692) (38.992, 178.1692) (40.1169, 178.3299) knots 0 0 0 1 1 1
  line L81 (40.1169, 178.3299) -> (32.973, 164.422)
  line L82 (32.973, 164.422) -> (30.8985, 163.8376)
  line L83 (30.8985, 163.8376) -> (36.8736, 175.4519)
  line L84 (36.8736, 175.4519) -> (31.9795, 175.6418)
  spline S263 degree 2 poles (31.9795, 175.6418) (31.6143, 175.6418) (30.767, 175.5104) knots 0 0 0 1 1 1
  line L85 (44.149, 176.4015) -> (46.6034, 178.3738)
  spline S264 degree 2 poles (46.6034, 178.3738) (48.3419, 178.2131) (51.103, 178.2131) knots 0 0 0 1 1 1
  spline S265 degree 2 poles (51.103, 178.2131) (52.374, 178.2131) (53.3236, 178.2131) knots 0 0 0 1 1 1
  line L86 (53.3236, 178.2131) -> (51.2345, 175.5834)
  line L87 (51.2345, 175.5834) -> (50.8692, 175.5834)
  spline S266 degree 2 poles (50.8692, 175.5834) (47.9912, 175.5834) (45.7122, 175.6857) knots 0 0 0 1 1 1
  line L88 (45.7122, 175.6857) -> (45.2593, 175.2182)
  line L89 (45.2593, 175.2182) -> (44.5727, 172.8223)
  spline S267 degree 2 poles (44.5727, 172.8223) (45.0986, 173.655) (46.6472, 173.655) knots 0 0 0 1 1 1
  spline S268 degree 2 poles (46.6472, 173.655) (48.5172, 173.655) (49.8612, 172.5739) knots 0 0 0 1 1 1
  spline S269 degree 2 poles (49.8612, 172.5739) (51.3367, 171.4198) (51.3367, 169.6082) knots 0 0 0 1 1 1
  spline S270 degree 2 poles (51.3367, 169.6082) (51.3367, 166.9932) (47.6844, 163.8376) (45.0402, 163.8376) knots 0 0 0 1 2 2 2
  spline S271 degree 2 poles (45.0402, 163.8376) (42.3083, 163.8376) (40.5698, 165.9998) knots 0 0 0 1 1 1
  line L90 (40.5698, 165.9998) -> (42.8342, 168.3665)
  spline S272 degree 2 poles (42.8342, 168.3665) (43.3601, 167.1539) (44.3828, 166.2043) knots 0 0 0 1 1 1
  spline S273 degree 2 poles (44.3828, 166.2043) (45.5661, 165.1524) (46.7495, 165.1524) knots 0 0 0 1 1 1
  spline S274 degree 2 poles (46.7495, 165.1524) (48.6779, 165.1524) (48.6779, 167.4753) knots 0 0 0 1 1 1
  spline S275 degree 2 poles (48.6779, 167.4753) (48.6779, 169.0239) (48.0789, 169.915) knots 0 0 0 1 1 1
  spline S276 degree 2 poles (48.0789, 169.915) (47.553, 170.7039) (45.5953, 171.6827) (44.6311, 171.6827) knots 0 0 0 1 2 2 2
  spline S277 degree 2 poles (44.6311, 171.6827) (44.3828, 171.6827) (43.5793, 171.3906) (43.4916, 171.3906) knots 0 0 0 1 2 2 2
  spline S278 degree 2 poles (43.4916, 171.3906) (42.9657, 171.3906) (42.9657, 171.7996) knots 0 0 0 1 1 1
  spline S279 degree 2 poles (42.9657, 171.7996) (42.9657, 172.1064) (43.0241, 172.2963) knots 0 0 0 1 1 1
  line L91 (43.0241, 172.2963) -> (44.149, 176.4015)
  point P0 (0, 0)
  point P1 (0, 133.9272)
  constraints: 1 midpoint, 1 vertical alignment, 2 other
extrude "Extrusion4" add sketch "Sketch4" along normal blind 2
body "Solid1"
